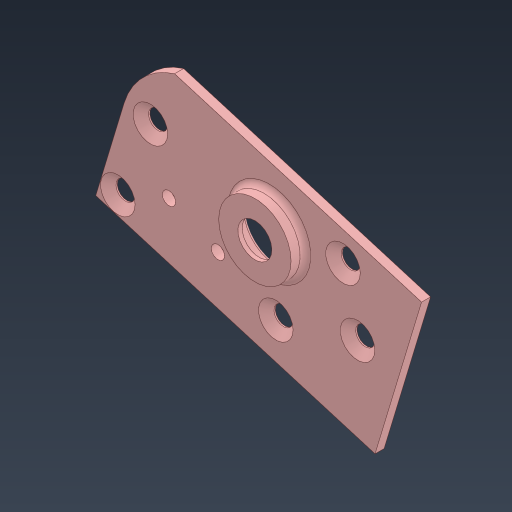
# Autodesk Inventor part: gearbox-left-wall
Saved by Autodesk Inventor 2023 (Build 270158000, 158)
## iProperties
Created: 2025-04-29
Part Number: gearbox-left-wall
Material: Generic
Document SubType Name: Modeling
Designer: szymo
Density: 1 g/cm^3
Appearance: Default(1)
Mass: 2.96908 g
Surface Area: 35.5974 cm^2
Volume: 2.96908 cm^3
Author: szymo
Autodesk Inventor part; units mm, degrees
ref_plane "YZ Plane" through (0, 0, 0) normal (1, 0, 0) x (0, 1, 0)
ref_plane "XZ Plane" through (0, 0, 0) normal (0, 1, 0) x (-1, 0, 0)
ref_plane "XY Plane" through (0, 0, 0) normal (0, 0, 1) x (1, 0, 0)
ref_plane "Work Plane1" through (-30.8963, -6.0374, 0) normal (0, 0, -1) x (0.9576375, -0.2879765, 0)
ref_plane "Work Plane2" through (-8.6276, -5.9719, 0.7) normal (0, 0, 1) x (0.9610211, 0.2764752, 0)
sketch "Sketch1" plane through (-30.8963, -6.0374, 0) normal (0, 0, -1) x (0.9576375, -0.2879765, 0)
  circle A0 centre (4.9956, -19.0263) radius 2.75 projected
  circle A1 centre (40.9685, -25.0739) radius 2.75 projected
  circle A2 centre (33.3568, -6.5487) radius 2.75 projected
  circle A3 centre (3.3273, -3.3164) radius 2.75 projected
  circle A4 centre (11.9462, -26.154) radius 2.25 projected
  line L0 (0, -18.4929) -> (0, 0) projected
  line L1 (0, 0) -> (54.8, 0) projected
  line L2 (54.8, 0) -> (54.8, -30.3429) projected
  line L3 (54.8, -30.3429) -> (6.3355, -30.3429) projected
  arc A5 (0, -18.4929) -> (6.3355, -30.3429) centre (14.25, -18.4929) ccw projected
  arc A6 (14.585, -3.786) -> (9.0794, -16.9358) centre (11.3142, -10.144) ccw projected
  arc A7 (9.0794, -16.9358) -> (18.5278, -21.7884) centre (14.25, -18.4929) ccw projected
  arc A8 (18.5278, -21.7884) -> (29.699, -9.4523) centre (28.2242, -19.3429) ccw projected
  arc A9 (29.699, -9.4523) -> (14.585, -3.786) centre (21.3244, -8.8) ccw projected
  circle A10 centre (28.2242, -19.3429) radius 6
  circle A11 centre (28.2242, -19.3429) radius 6 projected
  point P0 (27.8488, -14.679)
  dimension "d51" = 12
  constraints: 1 centre point
  measures "d51" diameter of A10
extrude "Extrusion1" add sketch "Sketch1" against normal up to surface (0.7 mm away) contours A0 | A1 | A2 | A3 | A4 | L0 L1 L2 L3 A5 | A9 A8 A7 A6
ref_plane "Work Plane3" through (-5.1842, -2.5285, 1.7) normal (0, 0, 1) x (0.9610211, 0.2764752, 0)
sketch "Sketch2" plane through (-30.8963, -6.0374, 0.7) normal (0, 0, 1) x (0.9576375, -0.2879765, 0)
  line L0 (54.8, 30.3429) -> (6.3355, 30.3429)
  arc A0 (6.3355, 30.3429) -> (0, 18.4929) centre (14.25, 18.4929) ccw
  line L1 (0, 18.4929) -> (0, 0)
  line L2 (0, -0.4836) -> (54.8, -0.4836)
  line L3 (54.8, 0) -> (54.8, 30.3429)
  circle A1 centre (28.2242, 19.3429) radius 6
  circle A2 centre (28.2242, 19.3429) radius 6 projected
  line L4 (54.8, 30.3429) -> (54.8, 0) projected
  line L5 (6.3355, 30.3429) -> (54.8, 30.3429) projected
  arc A3 (6.3355, 30.3429) -> (0, 18.4929) centre (14.25, 18.4929) ccw projected
  line L6 (0, 0) -> (0, 18.4929) projected
  line L7 (54.8, 0) -> (0, 0) projected
  dimension "d52" = 12
  constraints: 4 end point, 2 centre point, 2 point on circle, 1 concentric, 3 other
  measures "d52" diameter of A1
extrude "Extrusion2" add sketch "Sketch2" along normal up to surface (1 mm away)
sketch "Sketch4" plane through (-30.8963, -6.0374, 1.7) normal (0, 0, 1) x (0.9576375, -0.2879765, 0)
  circle A0 centre (3.3273, 3.3164) radius 2 projected
  circle A1 centre (4.9956, 19.0263) radius 2 projected
  circle A2 centre (40.9685, 25.0739) radius 2 projected
  arc A3 (32.8164, 8.4743) -> (35.3537, 6.4364) centre (33.3568, 6.5487) ccw projected
  circle A4 centre (46.8, 15.1715) radius 2 projected
  constraints: 5 coincident
hole "Hole1" at (2.9334, -9.372, 1.7) at (15.5574, 6.1764, 1.7) at (-20.6332, 10.7443, 1.7) at (-26.7549, -3.8196, 1.7) at (18.2902, -4.9859, 1.7) direction (0, 0, -1) diameter 3.6 end through all countersink diameter 6.5 countersink angle 90 clearance for "Countersunk Flat Head Screw ISO 2009/7046" size "M3" standard "ISO"
sketch "Sketch5" plane through (-30.8963, -6.0374, 0) normal (0, 0, -1) x (-0.9576375, 0.2879765, 0)
  circle A0 centre (-11.3142, 10.144) radius 1.25 projected
  circle A1 centre (-21.3244, 8.8) radius 1.25 projected
  circle A2 centre (-11.3142, 10.144) radius 1.25
  circle A3 centre (-21.3244, 8.8) radius 1.25
  point P0 (-27.8488, 14.679)
  dimension "d44" = 0
  dimension "d45" = 0
  constraints: 2 centre point
  measures "d44" radial gap between concentric circles of A3 A1
  measures "d45" radial gap between concentric circles of A2 A0
extrude "Extrusion4" cut sketch "Sketch5" against normal blind 7.25
sketch "Sketch9" plane through (-16.0911, 21.1957, 1.7) normal (0, 0, 1) x (0.9576375, -0.2879765, 0)
  circle A0 centre (21.8887, -11) radius 6
  circle A1 centre (21.8887, -11) radius 6.8
  point P0 (21.5133, -15.6639)
  dimension "d37" = 0.8
  dimension "d53" = 12
  constraints: 2 centre point, 1 other
  measures "d37" radial gap between concentric circles of A0 A1
  measures "d53" diameter of A0
extrude "Extrusion7" add sketch "Sketch9" along normal blind 1.9
sketch "Sketch10" plane through (1.7026, 4.3582, 3.6) normal (0, 0, 1) x (1, 0, 0)
  circle A0 centre (0, 0) radius 6.8 projected
  arc A1 (-2.3412, 1.8758) -> (0.9865, 2.8332) centre (0, 0) ccw projected
  circle A2 centre (0, 0) radius 3
  arc A3 (-2.4973, 2.0009) -> (1.0522, 3.022) centre (0, 0) ccw
  circle A4 centre (0, 0) radius 3.2
  point P0 (-1.7026, -4.3582)
  point P1 (1.0522, 3.022)
  dimension "d42" = 0.2
  constraints: 2 coincident, 2 point on circle, 1 centre point, 6 other
  measures "d42" radial gap between concentric circles of A1 A3
extrude "Extrusion8" add sketch "Sketch10" along normal blind 0.8 contours A0
fillet "Fillet5" radius 0.5 1 edges at (-4.0433, 6.0861, 0)
sketch "Sketch11" plane through (-7.941, -3.7511, 1.5) normal (0, 0, -1) x (-1, 0, 0)
  circle A0 centre (0, 0) radius 1.45 projected
  circle A1 centre (9.1991, 4.1698) radius 1.35 projected
  point P0 (-7.941, 3.7511)
extrude "Extrusion9" [suppressed]
fillet "Fillet6" radius 1 1 edges at (-4.8094, 6.3165, 1.7)
body "Solid1"
